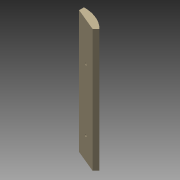
# Autodesk Inventor part: Foot2
Saved by Autodesk Inventor 2015 (Build 190159000, 159)
## iProperties
Created: 2015-09-26
Part Number: Foot2
Material: Generic
Document SubType Name: Modeling
Designer: Stefania
Density: 1 g/cm^3
Appearance: Beige
Author: Stefania
Autodesk Inventor part; units mm, degrees
ref_plane "YZ Plane" through (0, 0, 0) normal (1, 0, 0) x (0, 1, 0)
ref_plane "XZ Plane" through (0, 0, 0) normal (0, 1, 0) x (-1, 0, 0)
ref_plane "XY Plane" through (0, 0, 0) normal (0, 0, 1) x (1, 0, 0)
sketch "Sketch1" plane through (0, 0, 0) normal (0, 0, 1) x (1, 0, 0)
  line L0 (0, 0) -> (96.52, 0) construction
  line L1 (0, 83.82) -> (0, 96.52)
  line L2 (59.2697, 59.2697) -> (68.2499, 68.2499)
  line L3 (68.2499, 68.2499) -> (59.2697, 59.2697)
  line L4 (0, 83.82) -> (59.2697, 59.2697)
  arc A0 (68.2499, 68.2499) -> (0, 96.52) centre (0, 0) ccw
  constraints: 10 end point, 2 point on circle, 1 centre point, 1 coincident, 1 horizontal, 1 vertical
extrude "Extrusion1" add sketch "Sketch1" along normal mid plane 317.5
sketch "Sketch2" plane through (59.2697, 59.2697, -158.75) normal (-0.3827, -0.9239, 0) x (0.9239, -0.3827, 0)
  circle A0 centre (-32.0765, 57.912) radius 3.175
  line L0 (0, 0) -> (-64.1531, 0) projected
  circle A1 centre (-32.0765, 217.932) radius 3.175
  point P0 (-32.0765, 158.75)
  dimension "d5" = 6.35
  dimension "d6" = 57.912
  dimension "d7" = 6.35
  dimension "d8" = 160.02
  constraints: 2 centre point
  measures "d5" diameter of A0
  measures "d6" distance from line of L0 A0.centre
  measures "d7" diameter of A1
  measures "d8" distance of A1.centre A0.centre
extrude "Extrusion2" cut sketch "Sketch2" against normal blind 7.62
body "Solid1"
